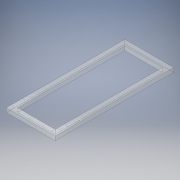
# Autodesk Inventor part: case_top_cover_slot
Saved by Autodesk Inventor 2019 (Build 230136000, 136)
## iProperties
Created: 2019-02-16
Part Number: case_top_cover_slot
Material: Acrylic, Clear
Document SubType Name: Modeling
Designer: suchanek
Density: 1.19 g/cm^3
Appearance: Transparent - Clear
Author: suchanek
Autodesk Inventor part; units mm, degrees
ref_plane "YZ Plane" through (0, 0, 0) normal (1, 0, 0) x (0, 1, 0)
ref_plane "XZ Plane" through (0, 0, 0) normal (0, 1, 0) x (-1, 0, 0)
ref_plane "XY Plane" through (0, 0, 0) normal (0, 0, 1) x (1, 0, 0)
sketch "Sketch1" plane through (0, 0, 0) normal (0, 1, 0) x (-1, 0, 0)
  line L0 (-27, 77) -> (27, 77)
  line L1 (27, 77) -> (27, -77)
  line L2 (27, -77) -> (-27, -77)
  line L3 (-27, -77) -> (-27, 77)
  line L4 (-27, 77) -> (27, -77) construction
  line L5 (27, 77) -> (-27, -77) construction
  line L6 (-35, 85) -> (35, 85)
  line L7 (35, 85) -> (35, -85)
  line L8 (35, -85) -> (-35, -85)
  line L9 (-35, -85) -> (-35, 85)
  line L10 (-35, 85) -> (35, -85) construction
  line L11 (35, 85) -> (-35, -85) construction
  point P0 (0, 0)
  point P1 (0, 0)
  dimension "d0" = 8
  dimension "d1" = 8
  dimension "d2" = 70
  dimension "d3" = 170
  constraints: 24 end point, 5 midpoint, 4 parallel, 2 horizontal, 2 perpendicular
  measures "d0" distance between parallel lines of L8 L2
  measures "d1" distance between parallel lines of L7 L1
  measures "d2" distance of L7.end L8.end
  measures "d3" distance of L6.end L7.end
extrude "Extrusion1" add sketch "Sketch1" along normal blind 6
equation "\"d1\" = d0"
body "Solid1"
